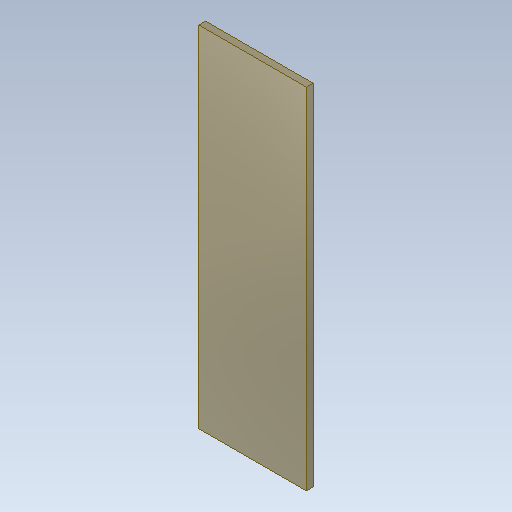
# Autodesk Inventor part: Nickel Strip
Saved by Autodesk Inventor 2020.1 (Build 241239000, 239)
## iProperties
Created: 2019-07-13
Part Number: Nickel Strip
Material: Generic
Document SubType Name: Modeling
Designer: Petar
Density: 1 g/cm^3
Appearance: Nickel
Author: Petar
Autodesk Inventor part; units mm, degrees
ref_plane "YZ Plane" through (0, 0, 0) normal (1, 0, 0) x (0, 1, 0)
ref_plane "XZ Plane" through (0, 0, 0) normal (0, 1, 0) x (-1, 0, 0)
ref_plane "XY Plane" through (0, 0, 0) normal (0, 0, 1) x (1, 0, 0)
sketch "Sketch1" plane through (0, 0, 0) normal (0, 0, 1) x (1, 0, 0)
  line L0 (-4, 3.835) -> (4, 3.835)
  line L1 (4, 3.835) -> (4, -22.165)
  line L2 (4, -22.165) -> (-4, -22.165)
  line L3 (-4, -22.165) -> (-4, 3.835)
  line L4 (-4, 3.835) -> (4, -22.165) construction
  line L5 (4, 3.835) -> (-4, -22.165) construction
  line L6 (-10.0664, -9.165) -> (174.6446, -9.165) construction
  line L7 (133.7834, -18.33) -> (159.5417, -18.33) construction
  line L8 (133.7834, 0) -> (159.5417, 0) construction
  line L9 (0, -12.831) -> (0, 12.8312) construction
  line L10 (0, -31.161) -> (0, -5.4988) construction
  point P0 (0, 0)
  point P1 (0, -9.165)
  dimension "d0" = 18.33
  dimension "d1" = 9.165
  dimension "d2" = 26
  dimension "d3" = 8
  constraints: 22 end point, 4 horizontal, 2 midpoint, 2 parallel, 2 vertical, 1 perpendicular, 1 point on line, 9 other
  measures "d0" distance between parallel lines of L7 L8
  measures "d1" distance between parallel lines of L7 L6
  measures "d2" distance of L0.end L1.end
  measures "d3" distance of L0.start L0.end
extrude "Extrusion1" add sketch "Sketch1" along normal blind 0.5
equation "\"d1\" = 0.5 * d0"
body "Solid1"
